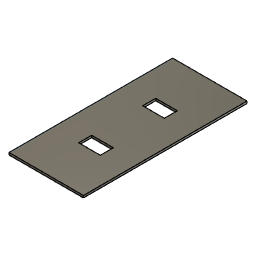
Bottom+cover+v1 (Autodesk Fusion 360 design; units mm, degrees)
Autodesk Fusion 360 part; units mm, degrees
sketch "Sketch1" plane through (0, 0, 0) normal (0, 1, 0) x (1, 0, 0)
  line L0 (0, 0) -> (170, 0)
  line L1 (170, 0) -> (170, -376)
  line L2 (170, -376) -> (0, -376)
  line L3 (0, -376) -> (0, 0)
  dimension "d1" = 170
  dimension "d2" = 376
  constraint horizontal L0
  constraint vertical L1
  constraint horizontal L2
  constraint vertical L3
  constraint coincident L0.start L3.end
  measures "d1" distance of L0.start L0.end
  measures "d2" distance of L0.start L2.end
extrude "Extrude1" add sketch "Sketch1" along normal blind 5
sketch "Sketch2" plane through (0, 0, 0) normal (-1, 0, 0) x (0, 0, 1)
  line L0 (0, 0) -> (376, 0)
  line L1 (376, 0) -> (376, 5)
  line L2 (376, 5) -> (0, 5)
  line L3 (0, 5) -> (0, 0)
extrude "Extrude2" cut 1 faces at (56.6667, 1.6667, 0) along direction (0, 0, 1) blind 3
extrude "Extrude3" cut 1 faces at (170, 1.6667, 127.3333) along direction (-1, 0, 0) blind 3
extrude "Extrude4" add 1 faces at (55.6667, 1.6667, 3) along direction (0, 0, -1) blind 3
extrude "Extrude5" add 1 faces at (167, 1.6667, 250.6667) along direction (1, 0, 0) blind 2
extrude "Extrude6" add 1 faces at (56.3333, 1.6667, 376) along direction (0, 0, 1) blind 2
extrude "Extrude7" add 1 faces at (169, 3.3333, 252) along direction (1, 0, 0) blind 3
sketch "Sketch3" plane through (0, 5, 0) normal (0, 1, 0) x (-1, 0, 0)
  line L0 (-172, 0) -> (0, 0)
  line L1 (0, 0) -> (0, 378)
  line L2 (0, 378) -> (-172, 378)
  line L3 (-172, 378) -> (-172, 0)
  line L4 (-61, 248) -> (-111, 248)
  line L5 (-111, 248) -> (-111, 278)
  line L6 (-111, 278) -> (-61, 278)
  line L7 (-61, 278) -> (-61, 248)
  line L8 (-61, 100) -> (-111, 100)
  line L9 (-111, 100) -> (-111, 130)
  line L10 (-111, 130) -> (-61, 130)
  line L11 (-61, 130) -> (-61, 100)
  dimension "d17" = 50
  dimension "d18" = 30
  dimension "d19" = 50
  dimension "d20" = 30
  dimension "d21" = 100
  dimension "d22" = 100
  dimension "d23" = 61
  dimension "d24" = 61
  constraint horizontal L4
  constraint vertical L5
  constraint horizontal L6
  constraint vertical L7
  constraint horizontal L8
  constraint vertical L9
  constraint horizontal L10
  constraint vertical L11
  measures "d17" distance of L4.start L4.end
  measures "d18" distance of L4.start L6.end
  measures "d19" distance of L8.start L8.end
  measures "d20" distance of L8.start L10.end
  measures "d21" vertical distance of L1.end L6.end
  measures "d22" vertical distance of L0.end L8.start
  measures "d23" horizontal distance of L1.end L6.end
  measures "d24" horizontal distance of L0.end L8.start
extrude "Extrude8" cut sketch "Sketch3" against normal blind 5 contours L4 L5 L6 L7 | L8 L9 L10 L11
